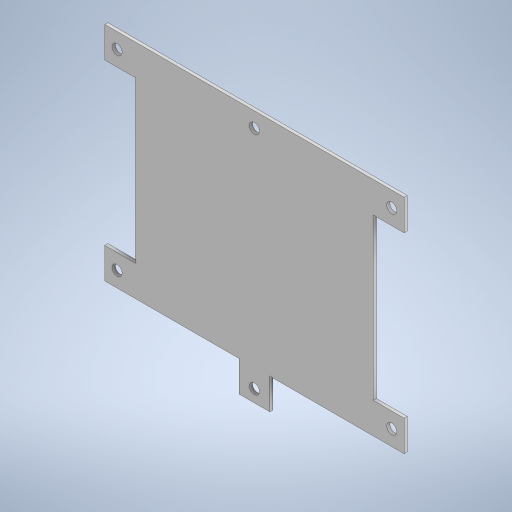
# Autodesk Inventor part: base
Saved by Autodesk Inventor 2023 (Build 270158000, 158)
## iProperties
Created: 2023-05-28
Part Number: base
Material: 一般
Document SubType Name: Sheet Metal
Designer: 310611102
Density: 1 g/cm^3
Sheet Metal Rule: Default_mm
Appearance: 預設
Author: 310611102
Autodesk Inventor part; units mm, degrees
ref_plane "YZ Plane" through (0, 0, 0) normal (1, 0, 0) x (0, 1, 0)
ref_plane "XZ Plane" through (0, 0, 0) normal (0, 1, 0) x (-1, 0, 0)
ref_plane "XY Plane" through (0, 0, 0) normal (0, 0, 1) x (1, 0, 0)
sketch "Sketch1" plane through (0, 0, 0) normal (0, 0, 1) x (1, 0, 0)
  line L0 (-38.5, 36) -> (38.5, 36)
  line L1 (38.5, 36) -> (38.5, -36)
  line L2 (38.5, -36) -> (-38.5, -36)
  line L3 (-38.5, -36) -> (-38.5, 36)
  line L4 (-38.5, 36) -> (38.5, -36) construction
  line L5 (38.5, 36) -> (-38.5, -36) construction
  circle A0 centre (0, 31.1) radius 1.6
  point P0 (0, 0)
  dimension "d0" = 72
  dimension "d1" = 77
  dimension "d24" = 3.2
  dimension "d25" = 4.9
  measures "d0" distance of L0.end L1.end
  measures "d1" distance of L0.start L0.end
  measures "d24" diameter of A0
  measures "d25" distance from line of L0 A0.centre
sketch "Sketch2" plane through (0, 0, 1) normal (0, 0, 1) x (1, 0, 0)
  line L0 (-38.5, 36) -> (38.5, 36)
  line L1 (-48.5, 26) -> (-38.5, 26)
  line L2 (-38.5, 26) -> (-38.5, 36)
  line L3 (-38.5, 36) -> (-48.5, 36)
  line L4 (-48.5, 36) -> (-48.5, 26)
  line L5 (-48.5, 26) -> (-38.5, 36) construction
  line L6 (-38.5, 26) -> (-48.5, 36) construction
  line L7 (0, 0) -> (0, 7.0571)
  line L8 (0, 0) -> (6.6312, 0)
  line L9 (-38.5, -36) -> (-38.5, 36)
  line L10 (48.5, 26) -> (38.5, 26)
  line L11 (38.5, 26) -> (38.5, 36)
  line L12 (38.5, 36) -> (48.5, 36)
  line L13 (48.5, 36) -> (48.5, 26)
  line L14 (48.5, 26) -> (38.5, 36) construction
  line L15 (38.5, 26) -> (48.5, 36) construction
  circle A0 centre (-44.5, 31) radius 1.6
  circle A1 centre (44.5, 31) radius 1.6
  line L16 (38.5, -36) -> (-38.5, -36)
  line L17 (-5, -46) -> (5, -46)
  line L18 (5, -46) -> (5, -36)
  line L19 (5, -36) -> (-5, -36)
  line L20 (-5, -36) -> (-5, -46)
  line L21 (-5, -46) -> (5, -36) construction
  line L22 (5, -46) -> (-5, -36) construction
  circle A2 centre (0, -42) radius 1.6
  line L23 (-48.5, -26) -> (-38.5, -26)
  line L24 (-38.5, -26) -> (-38.5, -36)
  line L25 (-38.5, -36) -> (-48.5, -36)
  line L26 (-48.5, -36) -> (-48.5, -26)
  line L27 (-48.5, -26) -> (-38.5, -36) construction
  line L28 (-38.5, -26) -> (-48.5, -36) construction
  line L29 (38.5, -26) -> (38.5, -36)
  line L30 (38.5, -36) -> (48.5, -36)
  line L31 (48.5, -36) -> (48.5, -26)
  line L32 (48.5, -26) -> (38.5, -36) construction
  line L33 (38.5, -26) -> (48.5, -36) construction
  line L34 (48.5, -26) -> (38.5, -26)
  circle A3 centre (-44.5, -31) radius 1.6
  circle A4 centre (44.5, -31) radius 1.6
  point P0 (-43.5, 31)
  point P1 (43.5, 31)
  point P2 (0, -41)
  point P3 (-38.5, -36)
  point P4 (-43.5, -31)
  point P5 (43.5, -31)
  dimension "d5" = 10
  dimension "d6" = 10
  dimension "d10" = 3.2
  dimension "d12" = 4
  dimension "d18" = 3.2
  dimension "d19" = 10
  dimension "d20" = 10
  dimension "d21" = 4
  dimension "d22" = 5
  measures "d5" distance of L2.end L3.end
  measures "d6" distance of L3.end L1.start
  measures "d10" diameter of A0
  measures "d12" distance from line of L4 A0.centre
  measures "d18" diameter of A2
  measures "d19" distance of L17.start L17.end
  measures "d20" distance of L19.end L17.start
  measures "d21" distance from line of L17 A2.centre
  measures "d22" distance from line of point (-43.5, 31) L0
extrude "Plate1" add sketch "Sketch1" along normal blind 1
sheet face with bend "Face2" sketch "Sketch2" thickness 1 toward (0, 0, -1) bend radius 1 relief straight relief width 1 relief depth 0.5
bend "Bend1"
equation "\"d2\" = 厚度"
equation "\"d13\" = 折彎半徑"
equation "\"d14\" = 折彎離隙寬度"
equation "\"d16\" = 最小剩餘"
equation "\"d15\" = 折彎離隙深度"
equation "\"d17\" = 轉移半徑"
equation "\"折彎半徑\" = 厚度"
equation "\"折彎離隙寬度\" = 厚度"
equation "\"折彎離隙深度\" = 0.5 * 厚度"
equation "\"轉角離隙大小\" = 4 * 厚度"
equation "\"最小剩餘\" = 2 * 厚度"
equation "\"轉移半徑\" = 折彎半徑"
equation "\"Jacobi半徑大小\" = 折彎半徑"
equation "\"間隙大小\" = 厚度"
equation "\"厚度\" = 1"
body "Solid1"
